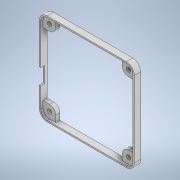
# Autodesk Inventor part: bumper
Saved by Autodesk Inventor 2020 (Build 240168000, 168)
## iProperties
Created: 2020-02-24
Part Number: bumper
Material: Generic
Document SubType Name: Modeling
Designer: Ray
Density: 1 g/cm^3
Appearance: Default
Author: Ray
Autodesk Inventor part; units mm, degrees
ref_plane "YZ Plane" through (0, 0, 0) normal (1, 0, 0) x (0, 1, 0)
ref_plane "XZ Plane" through (0, 0, 0) normal (0, 1, 0) x (-1, 0, 0)
ref_plane "XY Plane" through (0, 0, 0) normal (0, 0, 1) x (1, 0, 0)
sketch "Sketch1" plane through (0, 0, 0) normal (0, 0, 1) x (1, 0, 0)
  line L0 (36.83, -35.56) -> (-36.83, -35.56) construction
  line L1 (-36.83, -35.56) -> (-36.83, 35.56) construction
  line L2 (-36.83, 35.56) -> (36.83, 35.56) construction
  line L3 (36.83, 35.56) -> (36.83, -35.56) construction
  line L4 (36.83, -35.56) -> (-36.83, 35.56) construction
  line L5 (-36.83, -35.56) -> (36.83, 35.56) construction
  arc A0 (-31.75, 35.56) -> (-36.83, 30.48) centre (-31.75, 30.48) ccw construction
  arc A1 (36.83, 30.48) -> (31.75, 35.56) centre (31.75, 30.48) ccw construction
  arc A2 (-36.83, -30.48) -> (-31.75, -35.56) centre (-31.75, -30.48) ccw construction
  arc A3 (31.75, -35.56) -> (36.83, -30.48) centre (31.75, -30.48) ccw construction
  line L6 (31.75, -35.687) -> (-31.75, -35.687)
  line L7 (-36.957, -30.48) -> (-36.957, 30.48)
  line L8 (-31.75, 35.687) -> (31.75, 35.687)
  line L9 (36.957, 30.48) -> (36.957, -30.48)
  line L10 (36.957, -35.687) -> (-36.957, 35.687) construction
  line L11 (-36.957, -35.687) -> (36.957, 35.687) construction
  arc A4 (36.957, 30.48) -> (31.75, 35.687) centre (31.75, 30.48) ccw
  arc A5 (-31.75, 35.687) -> (-36.957, 30.48) centre (-31.75, 30.48) ccw
  arc A6 (-36.957, -30.48) -> (-31.75, -35.687) centre (-31.75, -30.48) ccw
  arc A7 (31.75, -35.687) -> (36.957, -30.48) centre (31.75, -30.48) ccw
  line L12 (-31.75, 36.887) -> (31.75, 36.887)
  line L13 (38.157, 30.48) -> (38.157, -30.48)
  line L14 (-31.75, -36.887) -> (31.75, -36.887)
  line L15 (-38.157, -30.48) -> (-38.157, 30.48)
  arc A8 (-31.75, 36.887) -> (-38.157, 30.48) centre (-31.75, 30.48) ccw
  arc A9 (38.157, 30.48) -> (31.75, 36.887) centre (31.75, 30.48) ccw
  arc A10 (31.75, -36.887) -> (38.157, -30.48) centre (31.75, -30.48) ccw
  arc A11 (-38.157, -30.48) -> (-31.75, -36.887) centre (-31.75, -30.48) ccw
  line L16 (-36.957, 25.4) -> (-31.75, 25.4)
  line L17 (-26.67, 35.687) -> (-26.67, 30.48)
  arc A12 (-31.75, 25.4) -> (-26.67, 30.48) centre (-31.75, 30.48) ccw
  circle A13 centre (-31.75, 30.48) radius 1.7145
  line L18 (0, 0) -> (78.9567, 0) construction
  line L19 (0, 0) -> (0, 57.9461) construction
  line L20 (36.957, 25.4) -> (31.75, 25.4)
  line L21 (26.67, 35.687) -> (26.67, 30.48)
  arc A14 (26.67, 30.48) -> (31.75, 25.4) centre (31.75, 30.48) ccw
  circle A15 centre (31.75, 30.48) radius 1.7145
  line L22 (-36.957, -25.4) -> (-31.75, -25.4)
  line L23 (-26.67, -35.687) -> (-26.67, -30.48)
  arc A16 (-26.67, -30.48) -> (-31.75, -25.4) centre (-31.75, -30.48) ccw
  circle A17 centre (-31.75, -30.48) radius 1.7145
  line L24 (36.957, -25.4) -> (31.75, -25.4)
  arc A18 (31.75, -25.4) -> (26.67, -30.48) centre (31.75, -30.48) ccw
  line L25 (26.67, -35.687) -> (26.67, -30.48)
  circle A19 centre (31.75, -30.48) radius 1.7145
  dimension "d0" = 73.66
  dimension "d1" = 71.12
  dimension "d2" = 5.08
  dimension "d4" = 0.127
  dimension "d5" = 0.127
  dimension "d7" = 1.2
  dimension "d12" = 10.16
  dimension "d13" = 10.16
  dimension "d14" = 3.429
  dimension "d22" = 1.2
  constraints: 52 end point, 32 point on circle, 20 centre point, 18 point on line, 18 symmetric about line, 10 tangent, 8 concentric, 5 coincident, 5 horizontal, 5 parallel, 5 vertical alignment, 4 midpoint, 4 perpendicular, 3 equal radius, 2 horizontal alignment, 2 vertical, 6 other
  measures "d0" distance of L1.end L2.end
  measures "d1" distance of L2.end L0.start
  measures "d2" distance from line of L2 A0.centre
  measures "d4" distance between parallel lines of L9 L3
  measures "d5" distance between parallel lines of L6 L0
  measures "d7" distance between parallel lines of L13 L9
  measures "d12" distance between parallel lines of L16 L2
  measures "d13" distance between parallel lines of L17 L1
  measures "d14" diameter of A13
  measures "d22" distance between parallel lines of L8 L12
extrude "Extrusion1" add sketch "Sketch1" along normal blind 5.08 contours L12 A9 L13 A10 L14 A11 L15 A8
extrude "Extrusion2" add sketch "Sketch1" along normal blind 3.302 contours L6 L25 A18 L24 L9 A7 | L6 A6 L7 L22 A16 L23 | L20 A14 L21 L8 A4 L9 | L7 A5 L8 L17 A12 L16
sketch "Sketch2" plane through (-38.157, -30.48, 0) normal (-1, 0, 0) x (0, 0, 1)
  line L0 (0, 0) -> (0, -6.407) projected
  line L1 (0, -6.407) -> (5.08, -6.407) projected
  line L2 (5.08, 0) -> (5.08, -6.407) projected
  line L3 (0, 0) -> (5.08, 0) projected
  line L4 (0, 60.96) -> (0, 0) projected
  line L5 (0, 0) -> (5.08, 0) projected
  line L6 (5.08, 60.96) -> (5.08, 0) projected
  line L7 (0, 60.96) -> (5.08, 60.96) projected
  line L8 (0, 67.367) -> (0, 60.96) projected
  line L9 (0, 60.96) -> (5.08, 60.96) projected
  line L10 (5.08, 67.367) -> (5.08, 60.96) projected
  line L11 (0, 67.367) -> (5.08, 67.367) projected
  line L12 (-16.8443, 22.549) -> (26.7617, 22.549) construction
  line L13 (5.08, 0) -> (5.08, 60.96) construction
  line L14 (2.032, 28.899) -> (5.08, 28.899)
  line L15 (5.08, 28.899) -> (5.08, 16.199) construction
  line L16 (5.08, 16.199) -> (2.032, 16.199)
  line L17 (2.032, 16.199) -> (2.032, 28.899)
  line L18 (2.032, 28.899) -> (5.08, 16.199) construction
  line L19 (5.08, 28.899) -> (2.032, 16.199) construction
  point P0 (0, 30.48)
  point P1 (3.556, 22.549)
  dimension "d17" = 28.956
  dimension "d18" = 12.7
  dimension "d19" = 3.048
  constraints: 14 end point, 2 horizontal, 2 midpoint, 2 parallel, 2 point on line, 1 perpendicular
  measures "d17" distance between parallel lines of L1 L12
  measures "d18" distance between parallel lines of L16 L14
  measures "d19" distance of L14.start L14.end
extrude "Extrusion3" cut sketch "Sketch2" against normal blind 2.54 contours L16 L17 L14 L6
body "Solid1"
